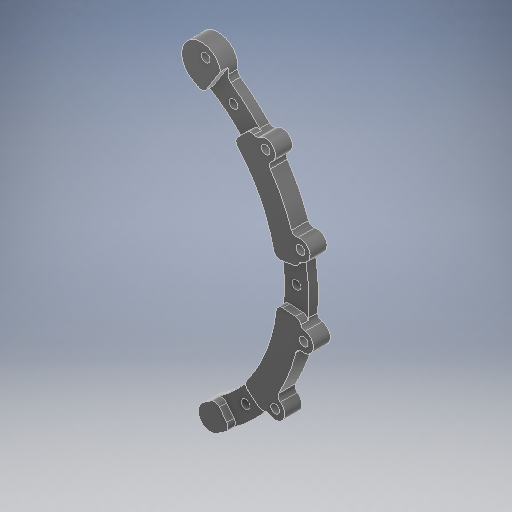
# Autodesk Inventor part: Robert
Saved by Autodesk Inventor 2026.1 (Build 301233000, 233)
## iProperties
Created: 2025-10-13
Part Number: Robert
Material: Plastic, Opaque Black
Document SubType Name: Modeling
Designer: Teddy
Density: 0.952 g/cm^3
Appearance: Smooth - Black
Author: Teddy
Autodesk Inventor part; units mm, degrees
ref_plane "YZ Plane" through (0, 0, 0) normal (1, 0, 0) x (0, 1, 0)
ref_plane "XZ Plane" through (0, 0, 0) normal (0, 1, 0) x (-1, 0, 0)
ref_plane "Work Plane1" through (0, 0, 0) normal (0, 0, 1) x (1, 0, 0)
sketch "Sketch1" plane through (0, 0, 0) normal (0, 0, 1) x (1, 0, 0)
  circle A0 centre (33.02, 0) radius 2.286
  circle A1 centre (0, 20.32) radius 2.286
  circle A2 centre (0, -20.32) radius 2.286
  circle A3 centre (-33.02, 0) radius 2.286
  circle A4 centre (-33.02, 0) radius 2.286
  circle A5 centre (33.02, 0) radius 2.286
  circle A6 centre (0, 20.32) radius 2.286
  circle A7 centre (0, -20.32) radius 2.286
  arc A8 (26.367455, -11.644455) -> (27.81191, -10.2) centre (26.367455, -10.2) ccw
  line L0 (26.367455, -11.644455) -> (25.45, -11.644455)
  arc A9 (25.45, -11.644455) -> (23.594455, -13.5) centre (25.45, -13.5) ccw
  line L1 (23.594455, -13.5) -> (23.594455, -14.217455)
  arc A10 (22.452, -15.629987) -> (23.594455, -14.217455) centre (22.15, -14.217455) ccw
  line L2 (22.452, -15.629987) -> (22.452, -15.827)
  line L3 (22.452, -15.827) -> (21.448, -15.827)
  line L4 (21.448, -15.827) -> (21.448, -15.66191)
  line L5 (21.448, -15.66191) -> (-22.15, -15.66191)
  arc A11 (-23.594455, -14.217455) -> (-22.15, -15.66191) centre (-22.15, -14.217455) ccw
  line L6 (-23.594455, -14.217455) -> (-23.594455, -13.5)
  arc A12 (-23.594455, -13.5) -> (-25.45, -11.644455) centre (-25.45, -13.5) ccw
  line L7 (-25.45, -11.644455) -> (-26.367455, -11.644455)
  arc A13 (-27.81191, -10.2) -> (-26.367455, -11.644455) centre (-26.367455, -10.2) ccw
  line L8 (-27.81191, -10.2) -> (-27.81191, 10.2)
  arc A14 (-26.367455, 11.644455) -> (-27.81191, 10.2) centre (-26.367455, 10.2) ccw
  line L9 (-26.367455, 11.644455) -> (-25.45, 11.644455)
  arc A15 (-25.45, 11.644455) -> (-23.594455, 13.5) centre (-25.45, 13.5) ccw
  line L10 (-23.594455, 13.5) -> (-23.594455, 14.217455)
  arc A16 (-22.15, 15.66191) -> (-23.594455, 14.217455) centre (-22.15, 14.217455) ccw
  line L11 (-22.15, 15.66191) -> (21.448, 15.66191)
  line L12 (21.448, 15.66191) -> (21.448, 15.827)
  line L13 (21.448, 15.827) -> (22.452, 15.827)
  line L14 (22.452, 15.827) -> (22.452, 15.629987)
  arc A17 (23.594455, 14.217455) -> (22.452, 15.629987) centre (22.15, 14.217455) ccw
  line L15 (23.594455, 14.217455) -> (23.594455, 13.5)
  arc A18 (23.594455, 13.5) -> (25.45, 11.644455) centre (25.45, 13.5) ccw
  line L16 (25.45, 11.644455) -> (26.367455, 11.644455)
  arc A19 (27.81191, 10.2) -> (26.367455, 11.644455) centre (26.367455, 10.2) ccw
  line L17 (27.81191, 10.2) -> (27.81191, -10.2)
  arc A20 (26.430088, -16.22496) -> (27.718677, -15.316229) centre (25.05, -12.9) ccw
  line L18 (27.718677, -15.316229) -> (37.72725, -4.26196)
  arc A21 (37.72725, -4.26196) -> (37.72725, 4.26196) centre (33.02, 0) ccw
  line L19 (37.72725, 4.26196) -> (27.718677, 15.316229)
  arc A22 (27.718677, 15.316229) -> (26.430088, 16.22496) centre (25.05, 12.9) ccw
  line L20 (26.430088, 16.22496) -> (2.434322, 26.18486)
  arc A23 (2.434322, 26.18486) -> (-2.434322, 26.18486) centre (0, 20.32) ccw
  line L21 (-2.434322, 26.18486) -> (-26.430088, 16.22496)
  arc A24 (-26.430088, 16.22496) -> (-27.718677, 15.316229) centre (-25.05, 12.9) ccw
  line L22 (-27.718677, 15.316229) -> (-37.72725, 4.26196)
  arc A25 (-37.72725, 4.26196) -> (-37.72725, -4.26196) centre (-33.02, 0) ccw
  line L23 (-37.72725, -4.26196) -> (-27.718677, -15.316229)
  arc A26 (-27.718677, -15.316229) -> (-26.430088, -16.22496) centre (-25.05, -12.9) ccw
  line L24 (-26.430088, -16.22496) -> (-2.434322, -26.18486)
  arc A27 (-2.434322, -26.18486) -> (2.434322, -26.18486) centre (0, -20.32) ccw
  line L25 (2.434322, -26.18486) -> (26.430088, -16.22496)
  circle A28 centre (28.397472, 78.830247) radius 3.9624 construction
  circle A29 centre (56.907559, 55.299166) radius 3.9624 construction
  circle A30 centre (73.381866, 22.206357) radius 3.9624 construction
  circle A31 centre (74.971837, -14.726133) radius 3.9624 construction
  circle A32 centre (61.402551, -49.11234) radius 3.9624 construction
  circle A33 centre (35.02026, -75.006578) radius 3.9624 construction
  circle A34 centre (-62.186251, 61.513849) radius 2.1844
  circle A35 centre (-72.793316, -46.442309) radius 2.1844
  arc A36 (35.02026, -75.006578) -> (28.397472, 78.830247) centre (-12.7, 0) ccw construction
  arc A37 (38.42885, -80.364191) -> (31.333006, 84.460978) centre (-12.7, 0) ccw
  arc A38 (31.61167, -69.648966) -> (25.461938, 73.199515) centre (-12.7, 0) ccw
  arc A39 (31.61167, -69.648966) -> (38.42885, -80.364191) centre (35.02026, -75.006578) ccw
  arc A40 (31.333006, 84.460978) -> (25.461938, 73.199515) centre (28.397472, 78.830247) ccw
  circle A41 centre (28.397472, 78.830247) radius 2.286
  circle A42 centre (56.907559, 55.299166) radius 2.286
  circle A43 centre (73.381866, 22.206357) radius 2.286
  circle A44 centre (74.971837, -14.726133) radius 2.286
  circle A45 centre (61.402551, -49.11234) radius 2.286
  circle A46 centre (35.02026, -75.006578) radius 2.286
  arc A47 (39.792286, -82.507236) -> (32.507219, 86.713271) centre (-12.7, 0) ccw construction
  circle A48 centre (32.507219, 86.713271) radius 2.286
  circle A49 centre (63.868315, 60.829082) radius 2.286
  circle A50 centre (81.990053, 24.426993) radius 2.286
  circle A51 centre (83.739021, -16.198746) radius 2.286
  circle A52 centre (68.812806, -54.023575) radius 2.286
  circle A53 centre (39.792286, -82.507236) radius 2.286
  line L26 (28.397472, 78.830247) -> (32.507219, 86.713271) construction
  arc A54 (40.079146, 79.290127) -> (25.461938, 73.199515) centre (30.229245, 82.343823) ccw
  arc A55 (64.502166, 55.788781) -> (59.101919, 62.586316) centre (63.868315, 60.829082) ccw
  arc A56 (56.973664, 64.947232) -> (60.606115, 64.723239) centre (58.907984, 66.750334) ccw
  arc A57 (66.923887, 56.770773) -> (66.320644, 53.181766) centre (68.514459, 54.658228) ccw
  arc A58 (77.366479, 30.993417) -> (80.593781, 29.311337) centre (79.866955, 31.853873) ccw
  arc A59 (80.519029, 19.564638) -> (78.350465, 27.970973) centre (81.990053, 24.426993) ccw
  arc A60 (83.130794, 19.476729) -> (81.119924, 16.443369) centre (83.724605, 16.899879) ccw
  arc A61 (82.185981, -8.319442) -> (84.450105, -11.16876) centre (84.820258, -8.550411) ccw
  arc A62 (80.417476, -20.042409) -> (81.855558, -11.480805) centre (83.739021, -16.198746) ccw
  arc A63 (82.767686, -21.185018) -> (79.696886, -23.138235) centre (82.26206, -23.780612) ccw
  arc A64 (70.598835, -46.193794) -> (71.508293, -49.717678) centre (72.911424, -47.476252) ccw
  arc A65 (64.215065, -56.183941) -> (69.011137, -48.947448) centre (68.812806, -54.023575) ccw
  arc A66 (65.897348, -58.183683) -> (62.297587, -58.719029) centre (64.379712, -60.349219) ccw
  point P0 (0, 0)
  point P1 (70.598835, -46.193794)
  point P2 (62.297587, -58.719029)
  point P3 (82.185981, -8.319442)
  point P4 (79.696886, -23.138235)
  point P5 (77.366479, 30.993417)
  dimension "d0" = 12.7
  dimension "d3" = 4.572
  dimension "d4" = 4.572
  dimension "d5" = 4.572
  dimension "d6" = 4.572
  dimension "d7" = 4.572
  dimension "d8" = 4.572
  dimension "d26" = 8.89
  dimension "d29" = 120
  dimension "d32" = 5.08
  dimension "d35" = 72
  constraints: 55 point on circle, 31 centre point, 9 tangent, 8 coincident, 2 end point, 1 equal radius, 1 line through centre, 1 point on line, 50 other
  measures "d0" diameter of A39
  measures "d3" diameter of A41
  measures "d4" diameter of A42
  measures "d5" diameter of A43
  measures "d6" diameter of A44
  measures "d7" diameter of A45
  measures "d8" diameter of A46
  measures "d26" radial gap between concentric circles of A36 A47
  measures "d32" radius of A55
extrude "Extrusion1" add sketch "Sketch1" along normal blind 8.89 contours A39 A38 A40 A37 | A37 A65 A66 | A37 A65 | A54 A37 A40 | A37 A64 A65 | A56 A55 A37 | A37 A62 A63 | A55 A37 | A37 A62 | A55 A57 A37 | A37 A61 A62 | A58 A59 A37 | A37 A59 A60 | A59 A37 | A41 | A42 | A43 | A44 | A45 | A46
fillet "Fillet2" radius 3.175 1 edges at (40.0791, 79.2901, 4.445)
sketch "Sketch2" plane through (0, 0, 8.89) normal (0, 0, 1) x (1, 0, 0)
  arc A0 (31.61167, -69.648966) -> (25.461938, 73.199515) centre (-12.7, 0) ccw
  arc A1 (38.42885, -80.364191) -> (62.297587, -58.719029) centre (-12.7, 0) ccw
  line L0 (31.258321, 69.872516) -> (38.02114, 80.622134)
  line L1 (46.99519, 57.017426) -> (56.179065, 65.789337)
  line L2 (68.639257, 14.08644) -> (81.152989, 16.253585)
  line L3 (69.616083, -6.210067) -> (82.280096, -7.165462)
  line L4 (52.194852, -51.021179) -> (62.178675, -58.870592)
  line L5 (37.765232, -65.328117) -> (45.529113, -75.378597)
  arc A2 (82.185981, -8.319442) -> (81.119924, 16.443369) centre (-12.7, 0) ccw
  line L6 (38.02114, 80.622134) -> (40.34982, 84.323612)
  arc A3 (40.466625, 81.102188) -> (25.461938, 73.199515) centre (30.229245, 82.343823) ccw
  arc A4 (56.973664, 64.947232) -> (40.079146, 79.290127) centre (-12.7, 0) ccw
  arc A5 (40.466625, 81.102188) -> (41.8018, 78.116043) centre (43.618527, 80.719912) ccw
  point P0 (0, 0)
  point P1 (37.765232, -65.328117)
  point P2 (45.529113, -75.378597)
  point P3 (62.178675, -58.870592)
  point P4 (52.194852, -51.021179)
  point P5 (69.616083, -6.210067)
  point P6 (82.265803, -7.352469)
  point P7 (81.184811, 16.068751)
  point P8 (68.639257, 14.08644)
  dimension "d10" = 20.32
  dimension "d14" = 96
  dimension "d38" = 7.51208
  constraints: 14 end point, 5 point on circle, 4 line through centre, 1 collinear, 13 other
  measures "d10" distance of L0.start L1.start
  measures "d38" distance from line of L0 A3.centre
extrude "Extrusion2" cut sketch "Sketch2" against normal blind 3.81 contours A0 L4 A1 L5 | A0 L2 A2 L3 | A0 L0 L6 A3 A5 A4 L1
sketch "Sketch3" plane through (0, 0, 5.08) normal (0, 0, 1) x (1, 0, 0)
  circle A0 centre (43.15884, 69.159236) radius 2.286
  circle A1 centre (76.119527, 3.781747) radius 2.286
  circle A2 centre (49.54225, -63.475289) radius 2.286
  arc A3 (35.02026, -75.006578) -> (28.397472, 78.830247) centre (-12.7, 0) ccw construction
  line L0 (56.179065, 65.789337) -> (46.99519, 57.017426)
  line L1 (68.639257, 14.08644) -> (81.152989, 16.253585)
  line L2 (52.194852, -51.021179) -> (62.178675, -58.870592)
  point P0 (0, 0)
  point P1 (73.381866, 22.206357)
  dimension "d18" = 4.572
  dimension "d19" = 11.43
  dimension "d20" = 11.43
  dimension "d21" = 11.43
  constraints: 6 point on circle, 4 centre point, 2 equal radius
  measures "d18" diameter of A2
  measures "d19" distance from line of L0 A0.centre
  measures "d20" distance from line of A1.centre L1
  measures "d21" distance from line of L2 A2.centre
extrude "Extrusion3" cut sketch "Sketch3" against normal through all
fillet "Fillet1" radius 3.175 11 edges at (31.2583, 69.8725, 6.985) (56.1791, 65.7893, 6.985) (45.5291, -75.3786, 6.985) (37.7652, -65.3281, 6.985) (52.1949, -51.0212, 6.985) (62.1787, -58.8706, 6.985) (82.2801, -7.1655, 6.985) (69.6161, -6.2101, 6.985) (81.153, 16.2536, 6.985) (68.6393, 14.0864, 6.985) (46.9952, 57.0174, 6.985)
body "Solid1"
